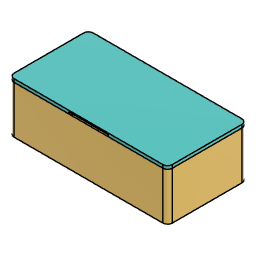
enclosure w_ snap fit lid v2 v24 (Autodesk Fusion 360 design; units mm, degrees)
Autodesk Fusion 360 part; units mm, degrees
sketch "base" plane through (0, 0, 0) normal (0, 0, 1) x (0, -1, 0) in component "base"
  line L0 (0, 0) -> (0, 100)
  line L1 (0, 100) -> (-50, 100)
  line L2 (-50, 100) -> (-50, 0)
  line L3 (-50, 0) -> (0, 0)
  dimension "d8" = 100
  dimension "d9" = 50
  constraint coincident L0.start L3.end
  measures "d8" distance of L0.start L0.end
  measures "d9" distance of L0.start L2.end
extrude "Extrude1" add sketch "base" along normal blind 30 makes body 1 in component "base"
fillet "Fillet1" radius 3 4 edges at (0, 0, 15) (0, 50, 15) (100, 50, 15) (100, 0, 15) on bodies 1 in component "base"
shell "Shell1" thickness 2 removed faces 1 at (34.3333, 33.3333, 30) on bodies 1 in component "base"
sketch "lip" plane through (0, 48, 0) normal (0, -1, 0) x (1, 0, 0) in component "base"
  line L0 (97, 2) -> (97, 30)
  line L1 (97, 30) -> (3, 30)
  line L2 (3, 30) -> (3, 2)
  line L3 (3, 2) -> (97, 2)
  line L4 (12.5, 30) -> (87.5, 30)
  line L5 (87.5, 30) -> (87.5, 25)
  line L6 (87.5, 25) -> (12.5, 25)
  line L7 (12.5, 25) -> (12.5, 30)
  line L8 (12.5, 27.5) -> (87.5, 27.5) construction
  dimension "d17" = 5
  dimension "d18" = 75
  constraint horizontal L4
  constraint vertical L5
  constraint horizontal L6
  constraint vertical L7
  constraint coincident L1 L4.start
  constraint midpoint L1 L4
  constraint midpoint L7 L8.start
  constraint midpoint L5 L8.end
  measures "d17" distance of L4.start L6.end
  measures "d18" distance of L5.end L6.end
ref_plane "WorkPlane1" through (12.5, 48, 27.5) normal (1, 0, 0) x (0, 1, 0) in component "base"
sketch "bead profile" plane through (12.5, 48, 27.5) normal (1, 0, 0) x (0, 1, 0) in component "base"
  line L0 (0, 0) -> (0, 1) construction
  arc A0 (0, 1) -> (0, -1) centre (0, 0) ccw
  line L1 (0, 1) -> (0, -1)
  dimension "d75" = 1
  constraint coincident L0.start A0.centre
  constraint vertical L0
  constraint parallel L0 L1
  measures "d75" distance of L0.start L0.end
sweep "Sweep1" add profiles "bead profile" path "lip" along L8 section 1 separate body makes body 2 in component "base"
fillet "Fillet7" radius 1 1 faces at (87.5, 47.7733, 27.7444) on bodies 2 in component "base"
fillet "Fillet7" radius 1 1 faces at (12.5, 47.7733, 27.7444) on bodies 2 in component "base"
ref_plane "WorkPlane2" through (50, 25, 16) normal (0, -1, 0) x (1, 0, 0) in component "base"
mirror "Mirror1" about plane through (50, 25, 16) normal (0, -1, 0) of bodies 2 makes body 3 in component "base"
combine "Combine4" operation add target body 1 tool bodies 2 3 keep tools in component "base"
fillet "Fillet8" radius 0.4 8 edges at (50, 48, 26.5) (12.5, 48, 27.5) (50, 48, 28.5) (87.5, 48, 27.5) (50, 2, 26.5) (87.5, 2, 27.5) (50, 2, 28.5) (12.5, 2, 27.5) on bodies 1 in component "base"
sketch "base projection" plane through (0, 0, 30) normal (0, 0, 1) x (-1, 0, 0) in component "lid"
  arc A0 (-97, -2) -> (-98, -3) centre (-97, -3) ccw
  line L0 (-97, -2) -> (-3, -2)
  arc A1 (-2, -3) -> (-3, -2) centre (-3, -3) ccw
  line L1 (-2, -3) -> (-2, -47)
  arc A2 (-3, -48) -> (-2, -47) centre (-3, -47) ccw
  line L2 (-3, -48) -> (-97, -48)
  arc A3 (-98, -47) -> (-97, -48) centre (-97, -47) ccw
  line L3 (-98, -47) -> (-98, -3)
  arc A4 (-97, 0) -> (-100, -3) centre (-97, -3) ccw
  line L4 (-100, -3) -> (-100, -47)
  arc A5 (-100, -47) -> (-97, -50) centre (-97, -47) ccw
  line L5 (-97, -50) -> (-3, -50)
  arc A6 (-3, -50) -> (0, -47) centre (-3, -47) ccw
  line L6 (0, -47) -> (0, -3)
  arc A7 (0, -3) -> (-3, 0) centre (-3, -3) ccw
  line L7 (-3, 0) -> (-97, 0)
extrude "Extrude1'" add sketch "base projection" along normal blind 2 separate body contours A0 L0 A1 L1 A2 L2 A3 L3 | A4 L4 A5 L5 A6 L6 A7 L7 makes body 4 in component "lid"
sketch "lip (2)" plane through (0, 0, 30) normal (0, 0, -1) x (1, 0, 0) in component "lid"
  line L0 (97, 0) -> (3, 0)
  arc A0 (3, 0) -> (0, -3) centre (3, -3) ccw
  line L1 (0, -3) -> (0, -47)
  arc A1 (0, -47) -> (3, -50) centre (3, -47) ccw
  line L2 (3, -50) -> (97, -50)
  arc A2 (97, -50) -> (100, -47) centre (97, -47) ccw
  line L3 (100, -47) -> (100, -3)
  arc A3 (100, -3) -> (97, 0) centre (97, -3) ccw
  line L4 (97.8, -47) -> (97.8, -3)
  arc A4 (97.8, -3) -> (97, -2.2) centre (97, -3) ccw
  line L5 (97, -2.2) -> (3, -2.2)
  arc A5 (3, -2.2) -> (2.2, -3) centre (3, -3) ccw
  line L6 (2.2, -3) -> (2.2, -47)
  arc A6 (2.2, -47) -> (3, -47.8) centre (3, -47) ccw
  line L7 (3, -47.8) -> (97, -47.8)
  arc A7 (97, -47.8) -> (97.8, -47) centre (97, -47) ccw
extrude "Extrude2" add sketch "lip (2)" along normal blind 5 contours L4 A4 L5 A5 L6 A6 L7 A7 bodies 4 in component "lid"
sketch "bead path" plane through (0, 47.8, 0) normal (0, 1, 0) x (-1, 0, 0) in component "lid"
  line L0 (-3, 30) -> (-97, 30)
  line L1 (-97, 25) -> (-3, 25)
  line L2 (-3, 25) -> (-3, 30)
  line L3 (-87.5, 30) -> (-12.5, 30) construction
  line L4 (-12.5, 30) -> (-12.5, 25) construction
  line L5 (-12.5, 25) -> (-87.5, 25) construction
  line L6 (-87.5, 25) -> (-87.5, 30) construction
  line L7 (-50, 30) -> (-50, 25) construction
  line L8 (-87.5, 27.5) -> (-12.5, 27.5)
  line L9 (-3, 30) -> (-97, 30)
  dimension "d82" = 75
  dimension "d83" = 5
  constraint horizontal L3
  constraint vertical L4
  constraint horizontal L5
  constraint vertical L6
  constraint midpoint L3 L7.start
  constraint midpoint L5 L7.end
  constraint midpoint L6 L8.start
  constraint midpoint L4 L8.end
  constraint midpoint L3 L9
  measures "d82" distance of L3.start L3.end
  measures "d83" distance of L3.start L5.end
ref_plane "WorkPlane2" through (50, 47.8, 27.5) normal (-1, 0, 0) x (0, -1, 0) in component "lid"
sketch "bead profile (2)" plane through (50, 47.8, 27.5) normal (-1, 0, 0) x (0, -1, 0) in component "lid"
  line L0 (0, 2.5) -> (0, -2.5)
  line L1 (0, 0) -> (-0.2, 0) construction
  line L2 (-0.2, 0) -> (-0.2, 1.2) construction
  arc A0 (-0.2, -1.2) -> (-0.2, 1.2) centre (-0.2, 0) ccw
  line L3 (-0.2, 1.2) -> (-0.2, -1.2)
  dimension "d85" = 0.2
  dimension "d86" = 1.2
  constraint coincident L1.start origin
  constraint perpendicular L0 L1
  constraint perpendicular L1 L2
  constraint coincident L1.end L2.start
  constraint parallel L2 L3
  measures "d85" distance of L1.start L1.end
  measures "d86" distance of L1.end L2.end
sweep "Sweep1'" add kept parallel profiles "bead profile (2)" path "bead path" along L8 section 1 contours L0 A0 separate body makes body 5 in component "lid"
fillet "Fillet4" radius 1.2 1 edges at (87.5, 46.8, 27.5) on bodies 5 in component "lid"
fillet "Fillet4" radius 1.2 1 edges at (12.5, 46.8, 27.5) on bodies 5 in component "lid"
mirror "Mirror1'" about plane through (50, 25, 16) normal (0, -1, 0) of bodies 5 makes body 6 in component "lid"
combine "Combine1" operation cut target body 4 tool bodies 5 6 keep tools in component "lid"
fillet "Fillet5" radius 0.4 tangency weight 1.4029 6 faces at (62.1, 47.742, 28.6719) (13.5419, 47.1759, 26.6422) (86.4581, 47.1759, 26.6422) (62.1, 3.0711, 28.0411) (13.5419, 2.8241, 28.3578) (86.4581, 2.8241, 26.6422) on bodies 4 in component "lid"
sketch "lip inner wall" plane through (0, 0, 25) normal (0, 0, -1) x (1, 0, 0) in component "lid"
  arc A0 (97, -47.8) -> (97.8, -47) centre (97, -47) ccw
  line L0 (97.8, -47) -> (97.8, -3)
  arc A1 (97.8, -3) -> (97, -2.2) centre (97, -3) ccw
  line L1 (97, -2.2) -> (3, -2.2)
  arc A2 (3, -2.2) -> (2.2, -3) centre (3, -3) ccw
  line L2 (2.2, -3) -> (2.2, -47)
  arc A3 (2.2, -47) -> (3, -47.8) centre (3, -47) ccw
  line L3 (3, -47.8) -> (97, -47.8)
  line L4 (4.2, -45.8) -> (95.8, -45.8)
  line L5 (95.8, -45.8) -> (95.8, -4.2)
  line L6 (95.8, -4.2) -> (4.2, -4.2)
  line L7 (4.2, -4.2) -> (4.2, -45.8)
  dimension "d54" = -2
extrude "Extrude3" cut sketch "lip inner wall" against normal blind 5 contours L4 L5 L6 L7 bodies 4 in component "lid"
fillet "Fillet6" radius 3 4 edges at (95.8, 45.8, 27.5) (95.8, 4.2, 27.5) (4.2, 4.2, 27.5) (4.2, 45.8, 27.5) on bodies 4 in component "lid"
fillet "Fillet6" radius 1.5 4 edges at (50, 4.2, 30) (4.2, 25, 30) (50, 45.8, 30) (95.8, 25, 30) on bodies 4 in component "lid"
fillet "Fillet9" radius 0.4 8 edges at (50, 48, 30) (97.7071, 47.7071, 30) (98, 25, 30) (97.7071, 2.2929, 30) (50, 2, 30) (2.2929, 2.2929, 30) (2, 25, 30) (2.2929, 47.7071, 30) on bodies 1 in component "base"
fillet "Fillet7'" radius 0.4 16 edges at (50, 2.2, 25) (2.4343, 2.4343, 25) (2.2, 25, 25) (2.4343, 47.5657, 25) (50, 47.8, 25) (97.5657, 47.5657, 25) (97.8, 25, 25) (97.5657, 2.4343, 25) (5.0787, 44.9213, 25) (4.2, 25, 25) (5.0787, 5.0787, 25) (50, 4.2, 25) (94.9213, 5.0787, 25) (95.8, 25, 25) (94.9213, 44.9213, 25) (50, 45.8, 25) on bodies 4 in component "lid"
fillet "Fillet8'" radius 0.4 8 edges at (50, 2.2, 30) (97.5657, 2.4343, 30) (97.8, 25, 30) (97.5657, 47.5657, 30) (50, 47.8, 30) (2.4343, 47.5657, 30) (2.2, 25, 30) (2.4343, 2.4343, 30) on bodies 4 in component "lid"
sketch "notch path" plane through (0, 0, 0) normal (0, -1, 0) x (1, 0, 0) in component "lid"
  line L0 (3, 30) -> (97, 30)
  line L1 (97, 30) -> (97, 32)
  line L2 (97, 32) -> (3, 32)
  line L3 (3, 32) -> (3, 30)
  line L4 (37.5, 32) -> (62.5, 32) construction
  line L5 (62.5, 32) -> (62.5, 30) construction
  line L6 (62.5, 30) -> (37.5, 30) construction
  line L7 (37.5, 30) -> (37.5, 32) construction
  line L8 (37.5, 30) -> (62.5, 30)
  dimension "notch_length" = 25
  dimension "d108" = 2
  constraint horizontal L4
  constraint vertical L5
  constraint horizontal L6
  constraint vertical L7
  constraint midpoint L0 L6
  measures "notch_length" distance of L4.start L4.end
  measures "d108" distance of L4.start L6.end
ref_plane "WorkPlane3" through (37.5, 0, 30) normal (1, 0, 0) x (0, 1, 0) in component "lid"
sketch "notch profile" plane through (37.5, 0, 30) normal (1, 0, 0) x (0, 1, 0) in component "lid"
  line L0 (0, 0) -> (0, 1)
  arc A0 (2.2, -0.4) -> (1.8, 0) centre (1.8, -0.4) ccw
  line L1 (1.8, 0) -> (0, 0)
  line L2 (0, 1) -> (1.8, 0)
  dimension "d111" = 1
  constraint coincident L0.start L1.end
  constraint coincident A0.end L1.start
  measures "d111" distance of L0.start L0.end
sweep "Sweep2" add profiles "notch profile" path "notch path" along L8 section 1 separate body makes body 7 in component "lid"
ref_plane "WorkPlane4" through (50, 25, 31) normal (0, -1, 0) x (1, 0, 0) in component "lid"
mirror "Mirror2" about plane through (50, 25, 31) normal (0, -1, 0) of bodies 7 makes body 8 in component "lid"
combine "Combine2" operation cut target body 4 tool bodies 7 8 keep tools in component "lid"
fillet "Fillet10" radius 0.4 2 edges at (50, 0, 31) (50, 50, 31) on bodies 4 in component "lid"
fillet "Fillet11" radius 0.4 tangency weight 1.38743 2 edges at (50, 1.8, 30) (50, 48.2, 30) on bodies 4 in component "lid"
component "base" placed x (1, 0, 0) y (0, 1, 0) z (0, 0, 1) at (0, 0, 0)
component "lid" placed x (1, 0, 0) y (0, 1, 0) z (0, 0, 1) at (0, 0, 0)
hidden bodies 2 3 5 6 7 8
equation "base_width = 50 mm" comment "width of the base (short dimension)"
equation "base_length = 100 mm" comment "length of the base (long dimension, includes the snap features)"
equation "base_height = 30 mm" comment "height of the base"
equation "shell_thickness = 2 mm" comment "thickness of the shell"
equation "corner_fillet = 3 mm"
equation "snap_feature_gap = 0.2 mm" comment "gap between the base and lid"
equation "snap_bead_radius = 1 mm" comment "radius of the semi-circular bead that forms the snap feature"
equation "d8 = base_length"
equation "d9 = base_width"
equation "d10 = base_height"
equation "d13 = corner_fillet"
equation "d14 = shell_thickness"
equation "lip_height = snap_bead_radius * 5" comment "height of the vertical lip - the snap feature is centered on this lip"
equation "snap_bead_length = base_length * 0.75" comment "length of the snap features"
equation "d17 = lip_height"
equation "d18 = snap_bead_length"
equation "lid_thickness = 2 mm" comment "thickness of the lid in the z direction (i.e., height)"
equation "d34 = lid_thickness"
equation "d36 = -( shell_thickness + snap_feature_gap )"
equation "d37 = lip_height"
equation "d54 = -( snap_bead_radius * 2 )"
equation "d75 = snap_bead_radius"
equation "d77 = snap_bead_radius"
equation "d79 = snap_bead_radius"
equation "d81 = snap_bead_fillet"
equation "d82 = snap_bead_length"
equation "d83 = lip_height"
equation "d85 = snap_feature_gap"
equation "d86 = snap_bead_radius + snap_feature_gap"
equation "d92 = snap_bead_radius + snap_feature_gap"
equation "d94 = snap_bead_radius + snap_feature_gap"
equation "snap_bead_fillet = 2 * snap_feature_gap"
equation "d98 = corner_fillet"
equation "d100 = corner_fillet / 2"
equation "d102 = snap_bead_fillet"
equation "d104 = snap_bead_fillet"
equation "d106 = snap_bead_fillet"
equation "notch_length = snap_bead_length / 3"
equation "d108 = lid_thickness"
equation "d111 = lid_thickness / 2"
equation "d125 = snap_bead_fillet"
equation "d127 = snap_bead_fillet"
equation "d136 = 1.5 * base_height"
named bodies: "base", "bead, back", "bead, front", "lid", "notch, front", "notch, back"
